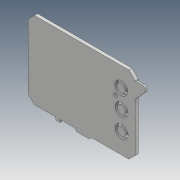
# Autodesk Inventor part: dibujo
Saved by Autodesk Inventor 2017 (Build 210142000, 142)
## iProperties
Created: 2020-06-11
Part Number: dibujo
Material: Generic
Document SubType Name: Modeling
Designer: c
Density: 1 g/cm^3
Appearance: Default
Author: c
Autodesk Inventor part; units mm, degrees
ref_plane "YZ Plane" through (0, 0, 0) normal (1, 0, 0) x (0, 1, 0)
ref_plane "Work Plane2" through (0, 0, 0) normal (0, -1, 0) x (1, 0, 0)
sketch "Sketch3" plane through (0, 0, 0) normal (0, -1, 0) x (1, 0, 0)
  line L0 (-2.9169, 8.7275) -> (27.2557, 8.7275)
  line L1 (29.2557, 6.7275) -> (29.2557, -13.939)
  line L2 (27.2557, -15.939) -> (-2.9169, -15.939)
  line L3 (-4.9169, -13.939) -> (-4.9169, 6.7275)
  line L4 (-4.9169, 6.7275) -> (-2.9169, 8.7275)
  line L5 (-4.9169, -13.939) -> (-2.9169, -15.939)
  line L6 (29.2557, -13.939) -> (27.2557, -15.939)
  line L7 (29.2557, 6.7275) -> (27.2557, 8.7275)
  point P0 (0, 0)
  point P1 (-4.9169, 8.7275)
  point P2 (29.2557, -15.939)
  point P3 (29.2557, 8.7275)
  point P4 (-4.9169, -15.939)
  dimension "d27" = 2
  dimension "d28" = 2
  dimension "d29" = 2
  dimension "d30" = 2
  dimension "d31" = 2
  dimension "d32" = 2
  dimension "d33" = 2
  dimension "d34" = 2
  constraints: 16 end point, 8 point on line, 2 parallel, 1 horizontal, 1 perpendicular
  measures "d27" distance of L3.end point (-4.917, 8.728)
  measures "d28" distance of L0.start point (-4.917, 8.728)
  measures "d29" distance of L3.start point (-4.917, -15.939)
  measures "d30" distance of L2.end point (-4.917, -15.939)
  measures "d31" distance of L1.end point (29.256, -15.939)
  measures "d32" distance of L2.start point (29.256, -15.939)
  measures "d33" distance of L1.start point (29.256, 8.728)
  measures "d34" distance of L0.end point (29.256, 8.728)
ref_plane "Work Plane1" through (0, 0, 0) normal (0, -1, 0) x (1, 0, 0)
sketch "Sketch4" plane through (0, 0, 0) normal (0, -1, 0) x (1, 0, 0)
  circle A0 centre (24.8305, 2.4994) radius 2.0487
  circle A1 centre (24.8305, 2.4994) radius 1.3931
  circle A2 centre (24.929, -3.3843) radius 2.0487
  circle A3 centre (24.929, -3.3843) radius 1.3931
  circle A4 centre (24.9456, -9.4318) radius 2.0487
  circle A5 centre (24.9456, -9.4318) radius 1.3931
  circle A6 centre (23.0022, -0.3984) radius 0.6003
  point P0 (0, 0)
  constraints: 7 centre point, 3 coincident
extrude "Extrusion2" add sketch "Sketch3" along normal blind 1
extrude "Extrusion3" cut sketch "Sketch4" along normal blind 2
sketch "Sketch6" plane through (0, -1, 0) normal (0, -1, 0) x (1, 0, 0)
  line L0 (-4.8835, 4.5825) -> (17.1165, 4.5825)
  line L1 (17.1165, 4.5825) -> (17.1165, 3.0825)
  line L2 (17.1165, 3.0825) -> (-4.8835, 3.0825)
  line L3 (-4.8835, 3.0825) -> (-4.8835, 4.5825)
  line L4 (17.1165, 3.0825) -> (15.6165, 3.0825)
  line L5 (15.6165, 3.0825) -> (15.6165, -11.4175)
  line L6 (15.6165, -11.4175) -> (17.1165, -11.4175)
  line L7 (17.1165, -11.4175) -> (17.1165, 3.0825)
  line L8 (-4.8835, 4.5825) -> (-3.3835, 4.5825)
  line L9 (-3.3835, 4.5825) -> (-3.3835, -11.4175)
  line L10 (-3.3835, -11.4175) -> (-4.8835, -11.4175)
  line L11 (-4.8835, -11.4175) -> (-4.8835, 4.5825)
  line L12 (-3.3835, -9.9175) -> (15.6165, -9.9175)
  line L13 (15.6165, -9.9175) -> (15.6165, -11.4175)
  line L14 (15.6165, -11.4175) -> (-3.3835, -11.4175)
  line L15 (-3.3835, -11.4175) -> (-3.3835, -9.9175)
  point P0 (0, 0)
  dimension "d50" = 1.5
  dimension "d51" = 1.5
  dimension "d52" = 1.5
  dimension "d53" = 1.5
  dimension "d54" = 22
  dimension "d59" = 16
  constraints: 32 end point, 8 parallel, 4 horizontal, 4 perpendicular, 2 point on line
  measures "d50" distance between parallel lines of L2 L0
  measures "d51" distance between parallel lines of L7 L5
  measures "d52" distance between parallel lines of L12 L14
  measures "d53" distance between parallel lines of L11 L9
  measures "d54" distance between parallel lines of L3 L1
  measures "d59" distance of L10.end L0.start
extrude "Extrusion4" add sketch "Sketch6" against normal blind 1.5 contours L0 L9 L2 L3 | L0 L1 L2 L9 | L2 L9 L10 L11 | L7 L6 L5 L2 | L12 L5 L14 L9
sketch "Sketch7" plane through (0, -1, 0) normal (0, -1, 0) x (1, 0, 0)
  line L0 (15.6165, 3.0825) -> (15.6165, -9.9175) projected
  line L1 (14.4114, -0.4847) -> (18.7497, -0.4847)
  line L2 (18.7497, -0.4847) -> (18.7497, -6.7959)
  line L3 (18.7497, -6.7959) -> (14.4114, -6.7959)
  line L4 (14.4114, -6.7959) -> (14.4114, -0.4847)
  arc A0 (15.9011, -3.328) -> (17.2497, -3.328) centre (16.5754, -4.3328) ccw
  line L5 (15.9011, -3.328) -> (15.3704, -1.6525)
  line L6 (15.3704, -1.6525) -> (17.7906, -1.6525)
  line L7 (17.7906, -1.6525) -> (17.2497, -3.328)
  line L8 (17.1165, -11.4175) -> (17.1165, 4.5825) projected
  point P0 (0, 0)
  constraints: 14 end point, 2 parallel, 2 point on circle, 1 centre point, 1 perpendicular
extrude "Extrusion5" add sketch "Sketch7" against normal blind 2 contours L1 L8 L6 L0 | L0 L6 L5 A0 L3 L4 L1 | L1 L2 L3 L8 A0 L7 L6 | L5 A0 L0 | L8 L3 L0 A0
sketch "Sketch8" plane through (0, 0, 0) normal (0, 1, 0) x (1, 0, 0)
  line L0 (14.4718, 6.0629) -> (17.9993, 6.0629)
  line L1 (17.9993, 6.0629) -> (17.9993, 1.2126)
  line L2 (17.9993, 1.2126) -> (14.4718, 1.2126)
  line L3 (14.4718, 1.2126) -> (14.4718, 6.0629)
  point P0 (0, 0)
  constraints: 8 end point, 2 parallel, 1 horizontal, 1 perpendicular
extrude "Extrusion6" add sketch "Sketch8" along normal blind 0.5
sketch "Sketch9" plane through (0, 0, 0) normal (0, 1, 0) x (1, 0, 0)
  line L0 (-4.7118, 10.795) -> (20.0243, 10.795) construction
  line L1 (20.0243, 10.795) -> (20.0243, -6.3237) construction
  line L2 (20.0243, -6.3237) -> (-4.7118, -6.3237) construction
  line L3 (-4.7118, -6.3237) -> (-4.7118, 10.795) construction
  line L4 (-7.5542, 17.4392) -> (33.1612, 17.4392) construction
  line L5 (33.1612, 17.4392) -> (33.1612, -10.738) construction
  line L6 (33.1612, -10.738) -> (-7.5542, -10.738) construction
  line L7 (-7.5542, -10.738) -> (-7.5542, 17.4392) construction
  point P0 (0, 0)
  constraints: 4 other
sketch "Sketch10" plane through (0, 0, 0) normal (0, 1, 0) x (1, 0, 0)
  line L0 (0.0858, 9.2478) -> (11.096, 9.2478)
  line L1 (12.096, 8.2478) -> (12.096, -1.6372)
  line L2 (11.096, -2.6372) -> (0.0858, -2.6372)
  line L3 (-0.9142, -1.6372) -> (-0.9142, 8.2478)
  arc A0 (0.0858, 9.2478) -> (-0.9142, 8.2478) centre (0.0858, 8.2478) ccw
  arc A1 (-0.9142, -1.6372) -> (0.0858, -2.6372) centre (0.0858, -1.6372) ccw
  arc A2 (11.096, -2.6372) -> (12.096, -1.6372) centre (11.096, -1.6372) ccw
  arc A3 (12.096, 8.2478) -> (11.096, 9.2478) centre (11.096, 8.2478) ccw
  point P0 (0, 0)
  dimension "d91" = 1
  constraints: 8 end point, 8 point on circle, 8 tangent, 4 centre point, 3 equal radius, 2 parallel, 1 horizontal, 1 perpendicular
  measures "d91" radius of A0
extrude "Extrusion7" cut sketch "Sketch10" against normal blind 0.5
sketch "Sketch11" plane through (0, 0, 0) normal (0, 1, 0) x (1, 0, 0)
  line L0 (3.9382, 16.7727) -> (5.2744, 16.7727)
  line L1 (5.2744, 16.7727) -> (5.2744, 15.2959)
  line L2 (5.2744, 15.2959) -> (3.9382, 15.2959)
  line L3 (3.9382, 15.2959) -> (3.9382, 16.7727)
  line L4 (27.2557, 15.939) -> (-2.9169, 15.939) projected
  line L5 (10.6317, 16.6774) -> (14.5822, 16.6774)
  line L6 (15.5822, 15.6774) -> (15.5822, 15.939)
  line L7 (15.5822, 15.939) -> (9.6317, 15.939)
  line L8 (9.6317, 15.939) -> (9.6317, 15.6774)
  line L9 (10.6317, 16.6774) -> (9.6317, 15.6774)
  line L10 (15.5822, 15.6774) -> (14.5822, 16.6774)
  line L11 (9.6895, 15.7352) -> (15.5244, 15.7352)
  point P0 (0, 0)
  point P1 (9.6317, 16.6774)
  point P2 (15.5822, 16.6774)
  constraints: 22 end point, 7 point on line, 5 parallel, 2 horizontal, 2 perpendicular
extrude "Extrusion8" add sketch "Sketch11" against normal blind 1 contours L0 L1 L4 L3 | L4 L1 L2 L3 | L9 L5 L10 L4 | L4 L10 L11 L9
sketch "Sketch12" plane through (0, 0, 0) normal (0, 1, 0) x (1, 0, 0)
  line L0 (28.9213, -6.7091) -> (31.5681, -6.7091)
  line L1 (32.3176, -5.047) -> (28.9213, -1.2028)
  line L2 (28.9213, -1.2028) -> (28.9213, -6.7091)
  arc A0 (31.5681, -6.7091) -> (32.3176, -5.047) centre (31.5681, -5.7091) ccw
  point P0 (0, 0)
  dimension "d96" = 1
  constraints: 6 end point, 2 point on circle, 2 tangent, 1 centre point, 1 horizontal, 1 perpendicular
  measures "d96" radius of A0
extrude "Extrusion9" add sketch "Sketch12" against normal blind 1
sketch "Sketch13" plane through (0, 0, 0) normal (0, 1, 0) x (1, 0, 0)
  line L0 (29.2557, -1.5814) -> (29.2557, 13.939) projected
  line L1 (29.2557, 0.5613) -> (34.1068, 0.5613)
  line L2 (34.1068, 0.5613) -> (34.1068, -7.7248)
  line L3 (34.1068, -7.7248) -> (29.2557, -7.7248)
  line L4 (29.2557, -7.7248) -> (29.2557, 0.5613)
  point P0 (0, 0)
  constraints: 8 end point, 2 parallel, 1 horizontal, 1 perpendicular, 1 point on line
extrude "Extrusion10" cut sketch "Sketch13" against normal blind 0.5
sketch "Sketch14" plane through (0, 0, 0) normal (0, 1, 0) x (1, 0, 0)
  point P0 (0, 0)
sketch "Sketch15" plane through (0, 0, 0) normal (0, 1, 0) x (1, 0, 0)
  line L0 (5.2744, 15.939) -> (27.2557, 15.939) projected
  line L1 (-2.0879, 17.695) -> (16.1478, 17.695)
  line L2 (16.1478, 17.695) -> (16.1478, 15.939)
  line L3 (16.1478, 15.939) -> (-2.0879, 15.939)
  line L4 (-2.0879, 15.939) -> (-2.0879, 17.695)
  point P0 (0, 0)
  constraints: 8 end point, 2 parallel, 1 horizontal, 1 perpendicular, 1 point on line
extrude "Extrusion11" cut sketch "Sketch15" against normal blind 0.5
equation "\"d28\" = d27"
equation "\"d29\" = d27"
equation "\"d30\" = d29"
equation "\"d31\" = d27"
equation "\"d32\" = d31"
equation "\"d33\" = d27"
equation "\"d34\" = d33"
body "Solid1"
